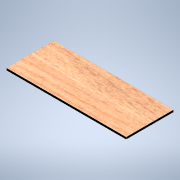
# Autodesk Inventor part: wood_front
Saved by Autodesk Inventor 2021 (Build 250183000, 183)
## iProperties
Created: 2021-08-17
Part Number: wood_front
Material: Generisch
Document SubType Name: Modeling
Designer: Tilman
Density: 1 g/cm^3
Appearance: Eloxiert - Schwarz
Author: Tilman
Autodesk Inventor part; units mm, degrees
ref_plane "YZ Plane" through (0, 0, 0) normal (1, 0, 0) x (0, 1, 0)
ref_plane "XZ Plane" through (0, 0, 0) normal (0, 1, 0) x (-1, 0, 0)
ref_plane "XY Plane" through (0, 0, 0) normal (0, 0, 1) x (1, 0, 0)
sketch "Skizze1" plane through (0, 0, 0) normal (0, 1, 0) x (-1, 0, 0)
  line L0 (0, 0) -> (-165.5, 0)
  line L1 (-165.5, 0) -> (-165.5, -65.5)
  line L2 (-165.5, -65.5) -> (0, -65.5)
  line L3 (0, -65.5) -> (0, 0)
  line L4 (-39.75, -43.25) -> (-57.75, -43.25)
  line L5 (-57.75, -43.25) -> (-57.75, -22.25)
  line L6 (-57.75, -22.25) -> (-39.75, -22.25)
  line L7 (-39.75, -22.25) -> (-39.75, -43.25)
  line L8 (-107.75, -22.25) -> (-125.75, -22.25)
  line L9 (-125.75, -22.25) -> (-125.75, -43.25)
  line L10 (-125.75, -43.25) -> (-107.75, -43.25)
  line L11 (-107.75, -43.25) -> (-107.75, -22.25)
  line L12 (-57.75, -32.75) -> (-107.75, -32.75) construction
  point P0 (-39.75, -32.75)
  point P1 (0, -32.75)
  point P2 (-125.75, -32.75)
  point P3 (-165.5, -32.75)
  point P4 (-82.75, -32.75)
  point P5 (-82.75, 0)
  dimension "d0" = 165.5
  dimension "d1" = 65.5
  dimension "d4" = 21
  dimension "d5" = 18
  dimension "d6" = 50
  constraints: 26 end point, 8 midpoint, 6 parallel, 3 horizontal, 3 perpendicular, 2 equal length, 2 horizontal alignment, 1 vertical alignment
  measures "d0" distance of L0.start L0.end
  measures "d1" distance of L2.end L0.start
  measures "d4" distance of L6.end L4.start
  measures "d5" distance of L4.start L4.end
  measures "d6" distance of L12.start L12.end
extrude "Extrusion1" add sketch "Skizze1" along normal blind 3 contours L3 L2 L1 L0 | L4 L5 L6 L7 | L11 L10 L9 L8
